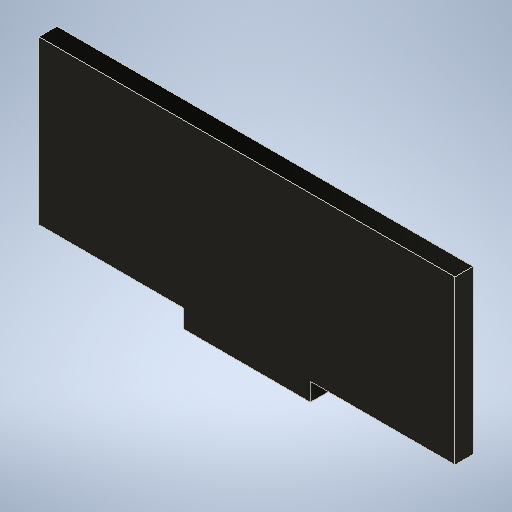
# Autodesk Inventor part: front
Saved by Autodesk Inventor 2025.3 (Build 293356030, 356C)
## iProperties
Created: 2026-06-25
Part Number: front
Material: Generic
Document SubType Name: Modeling
Designer: user
Density: 1 g/cm^3
Appearance: Gunmetal
Author: user
Autodesk Inventor part; units mm, degrees
ref_plane "YZ Plane" through (0, 0, 0) normal (1, 0, 0) x (0, 1, 0)
ref_plane "XZ Plane" through (0, 0, 0) normal (0, 1, 0) x (-1, 0, 0)
ref_plane "XY Plane" through (0, 0, 0) normal (0, 0, 1) x (1, 0, 0)
sketch "Sketch1" plane through (0, 0, 0) normal (0, 0, 1) x (1, 0, 0)
  line L0 (80, 0) -> (150, 0)
  line L1 (230, 10) -> (230, 100)
  line L2 (230, 100) -> (0, 100)
  line L3 (0, 100) -> (0, 10)
  line L4 (80, 0) -> (150, 0)
  line L5 (150, 0) -> (150, 10)
  line L6 (80, 10) -> (80, 0)
  line L7 (80, 10) -> (0, 10)
  line L8 (150, 10) -> (230, 10)
  dimension "d9" = 230
  dimension "d13" = 100
  dimension "d14" = 10
  constraints: 18 end point, 3 parallel, 2 equal length, 2 horizontal, 2 perpendicular
  measures "d9" distance of L2.end L1.end
  measures "d13" distance between parallel lines of L2 L0
  measures "d14" distance from line of L3.end L0
extrude "Extrusion1" add sketch "Sketch1" along normal blind 10
body "Solid1"
